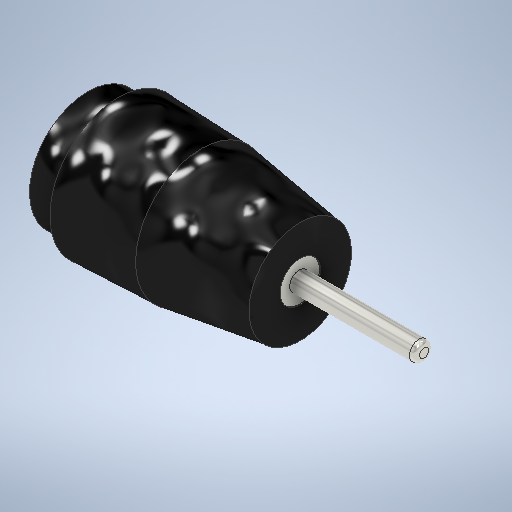
# Autodesk Inventor part: CT3149-0-Banana-Connector
Saved by Autodesk Inventor 2025 (Build 290162000, 162)
## iProperties
Created: 2026-01-19
Part Number: CT3149-0-Banana-Connector
Material: Generic
Document SubType Name: Modeling
Designer: tapen
Density: 1 g/cm^3
Appearance: Default
Author: tapen
Autodesk Inventor part; units mm, degrees
ref_plane "YZ Plane" through (0, 0, 0) normal (1, 0, 0) x (0, 1, 0)
ref_plane "XZ Plane" through (0, 0, 0) normal (0, 1, 0) x (-1, 0, 0)
ref_plane "XY Plane" through (0, 0, 0) normal (0, 0, 1) x (1, 0, 0)
sketch "Sketch1" plane through (0, 0, 0) normal (0, 0, 1) x (1, 0, 0)
  line L0 (0, 0) -> (0, 5.75)
  line L1 (0, 5.75) -> (3, 5.75)
  line L2 (3, 5.75) -> (3, 6.75)
  line L3 (20.9195, 5.0497) -> (20.9195, 0.95)
  line L4 (20.9195, 0.95) -> (32.6195, 0.95)
  line L5 (33.1195, 0.45) -> (33.1195, 0)
  line L6 (33.1195, 0) -> (0, 0)
  arc A0 (33.1195, 0.45) -> (32.6195, 0.95) centre (32.6195, 0.45) ccw
  line L7 (-7.1846, 0) -> (0, 0) construction
  line L8 (3, 6.75) -> (11.155, 6.4559)
  line L9 (11.155, 6.4559) -> (20.9195, 5.0497)
  point P0 (33.1195, 0.95)
  dimension "d0" = 5.75
  dimension "d1" = 3
  dimension "d2" = 1
  dimension "d3" = 18
  dimension "d5" = 12.2
  dimension "d6" = 0.5
  dimension "d11" = 0.95
  constraints: 21 end point, 3 horizontal, 3 vertical, 2 perpendicular, 2 point on circle, 2 point on line, 2 tangent, 1 centre point
  measures "d0" distance of L0.start L0.end
  measures "d1" distance of L0.end L1.end
  measures "d2" distance of L1.end L2.end
  measures "d3" distance of L3.start L2.end
  measures "d5" distance of L3.end point (33.12, 0.95)
  measures "d6" radius of A0
  measures "d11" distance from line of L3.end L6
revolve "Revolution1" add sketch "Sketch1" angle 360 about axis through (-7.1846, 0, 0) along (1, 0, 0)
sketch "Sketch2" plane through (0, 0, 0) normal (-1, 0, 0) x (0, 0, 1)
  circle A0 centre (0, 0) radius 2
  dimension "d8" = 4
  constraints: 1 centre point, 1 coincident
  measures "d8" diameter of A0
extrude "Extrusion1" cut sketch "Sketch2" against normal blind 20
sketch "Sketch3" plane through (20.9195, 0, 0) normal (1, 0, 0) x (0, 0, -1)
  circle A0 centre (0, 0) radius 0.45 projected
  circle A1 centre (0, 0) radius 2
  circle A2 centre (0, 0) radius 0.95 projected
  circle A3 centre (0, 0) radius 0.95
  dimension "d12" = 4
  constraints: 2 centre point, 2 coincident
  measures "d12" diameter of A1
extrude "Extrusion2" cut sketch "Sketch3" against normal blind 0.1 contours A1
body "Solid1"
